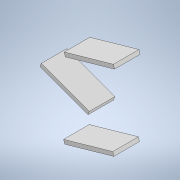
# Autodesk Inventor part: zigzags
Saved by Autodesk Inventor 2020 (Build 240168000, 168)
## iProperties
Created: 2020-12-28
Part Number: zigzags
Material: Generic
Document SubType Name: Modeling
Designer: solar
Density: 1 g/cm^3
Appearance: Default
Author: solar
Autodesk Inventor part; units mm, degrees
ref_plane "YZ Plane" through (0, 0, 0) normal (1, 0, 0) x (0, 1, 0)
ref_plane "XZ Plane" through (0, 0, 0) normal (0, 1, 0) x (-1, 0, 0)
ref_plane "XY Plane" through (0, 0, 0) normal (0, 0, 1) x (1, 0, 0)
sketch "Sketch1" plane through (0, 0, 0) normal (0, 0, 1) x (1, 0, 0)
  line L0 (-60, -100) -> (60, -100)
  line L1 (60, -100) -> (60, 100)
  line L2 (60, 100) -> (-60, 100)
  line L3 (-60, 100) -> (-60, -100)
  line L4 (-60, -100) -> (60, 100) construction
  line L5 (60, -100) -> (-60, 100) construction
  line L6 (-60, 68.3879) -> (-20, 68.3879)
  line L7 (60, 18.819) -> (20, 18.819)
  line L8 (-20, 68.3879) -> (-20, -101.8705)
  line L9 (-20, 68.3879) -> (-20, 105.2952)
  line L10 (20, 18.819) -> (20, 105.2952)
  line L11 (20, 18.819) -> (20, -103.7563)
  line L12 (56.9386, -47.8111) -> (-20, -69.7303)
  line L13 (56.9386, -47.8111) -> (58.5825, -53.5815)
  line L14 (58.5825, -53.5815) -> (-18.3561, -75.5007)
  line L15 (-18.3561, -75.5007) -> (-20, -69.7303)
  line L16 (20.1346, -11.7915) -> (-54.9978, 15.6882)
  line L17 (-54.9978, 15.6882) -> (-57.0588, 10.0532)
  line L18 (-57.0588, 10.0532) -> (18.0736, -17.4264)
  line L19 (18.0736, -17.4264) -> (20.1346, -11.7915)
  line L20 (20.1346, -11.7915) -> (-57.0588, 10.0532) construction
  line L21 (-54.9978, 15.6882) -> (18.0736, -17.4264) construction
  line L22 (-18.3561, 42.3147) -> (-18.3561, 2.3147)
  line L23 (57.9386, 71.0043) -> (-19, 49.0851)
  line L24 (57.9386, 71.0043) -> (59.5825, 65.2339)
  line L25 (59.5825, 65.2339) -> (-17.3561, 43.3147)
  line L26 (-17.3561, 43.3147) -> (-19, 49.0851)
  line L27 (18.0736, -17.4264) -> (18.0736, -57.4264)
  point P0 (0, 0)
  point P1 (-15.0354, 25.059)
  dimension "d0" = 120
  dimension "d1" = 200
  dimension "d2" = 40
  dimension "d3" = 40
  dimension "d4" = 80
  dimension "d5" = 6
  dimension "d6" = 80
  dimension "d7" = 6
  dimension "d8" = 40
  dimension "d9" = 15.902
  dimension "d10" = 80
  dimension "d11" = 6
  dimension "d12" = 39.8706
  dimension "d13" = 40
  constraints: 56 end point, 7 perpendicular, 5 parallel, 5 vertical, 3 point on line, 2 horizontal, 2 midpoint
  measures "d0" distance of L2.end L1.end
  measures "d1" distance of L1.end L0.end
  measures "d2" distance of L6.start L6.end
  measures "d3" distance of L7.start L7.end
  measures "d4" distance of L12.start L12.end
  measures "d5" distance of L12.start L13.end
  measures "d6" distance of L18.end L17.end
  measures "d7" distance of L17.end L16.end
  measures "d8" distance of L22.start L22.end
  measures "d9" angle of L2 L14
  measures "d10" distance of L23.start L23.end
  measures "d11" distance of L23.start L25.start
  measures "d12" distance from line of L12 L18.end
  measures "d13" distance of L18.end L27.end
extrude "Extrusion1" add sketch "Sketch1" along normal blind 40 contours L12 L11 L14 L15 | L11 L12 L13 L14 | L18 L17 L16 L8 | L8 L16 L11 L19 L18 | L11 L16 L19 | L23 L24 L25 L10 | L10 L25 L26 L23
body "Solid1"
